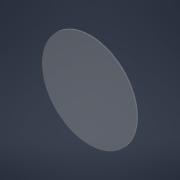
# Autodesk Inventor part: poly carbonate plate
Saved by Autodesk Inventor 2021 (Build 250183000, 183)
## iProperties
Created: 2022-05-21
Part Number: poly carbonate plate
Material: Polycarbonate, Clear
Document SubType Name: Modeling
Designer: techv
Mass: 126.54 g
Surface Area: 725.5 cm^2
Volume: 105.45 cm^3
Density: 1.2 g/cm^3
Appearance: Polycarbonate - Clear
Author: techv
Autodesk Inventor part; units mm, degrees
ref_plane "YZ Plane" through (0, 0, 0) normal (1, 0, 0) x (0, 1, 0)
ref_plane "XZ Plane" through (0, 0, 0) normal (0, 1, 0) x (-1, 0, 0)
ref_plane "XY Plane" through (0, 0, 0) normal (0, 0, 1) x (1, 0, 0)
sketch "Sketch1" plane through (0, 0, 0) normal (0, 0, 1) x (1, 0, 0)
  line L0 (-95, -92.5) -> (95, 92.5) construction
  line L1 (95, -92.5) -> (-95, 92.5) construction
  circle A0 centre (0, 0) radius 101
  dimension "d0" = 190
  dimension "d1" = 185
  dimension "d4" = 202
  constraints: 4 end point, 2 midpoint, 1 centre point, 1 coincident
  measures "d0" distance of L0.end L1.end
  measures "d1" distance of L1.end L0.start
  measures "d4" diameter of A0
extrude "Extrusion1" add sketch "Sketch1" along normal blind 3
body "Solid1"
